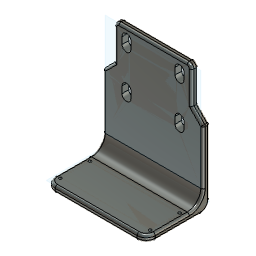
Polycase-Voltaic-Bracket v11 (Autodesk Fusion 360 design; units mm, degrees)
Autodesk Fusion 360 part; units mm, degrees
sketch "Sketch1" plane through (0, 0, 0) normal (0, 0, 1) x (1, 0, 0)
sketch "Sketch2" plane through (0, 0, 0) normal (0, 0, 1) x (1, 0, 0)
  line L0 (-101.7193, 55.502) -> (37.9807, 55.502)
  line L1 (37.9807, 55.502) -> (37.9807, -33.398)
  line L2 (37.9807, -33.398) -> (-101.7193, -33.398)
  line L3 (-101.7193, -33.398) -> (-101.7193, 55.502)
  dimension "d1" = 139.7
  dimension "d2" = 88.9
  constraint horizontal L0
  constraint vertical L1
  constraint horizontal L2
  constraint vertical L3
  measures "d1" distance of L0.start L0.end
  measures "d2" distance of L0.end L1.end
extrude "Extrude1" add sketch "Sketch2" along normal blind 9.525
sketch "Sketch3" plane through (0, 0, 9.525) normal (0, 0, 1) x (-1, 0, 0)
  line L0 (101.7193, 33.398) -> (-37.9807, 33.398)
  line L1 (-37.9807, 33.398) -> (-37.9807, -55.502)
  line L2 (-37.9807, -55.502) -> (101.7193, -55.502)
  line L3 (101.7193, -55.502) -> (101.7193, 33.398)
sketch "Sketch4" plane through (0, 0, 9.525) normal (0, 0, 1) x (-1, 0, 0)
  line L0 (-37.9807, -55.502) -> (101.7193, -55.502)
  line L1 (101.7193, -55.502) -> (101.7193, -45.977)
  line L2 (101.7193, -45.977) -> (-37.9807, -45.977)
  line L3 (-37.9807, -45.977) -> (-37.9807, -55.502)
  line L4 (101.7193, -55.502) -> (101.7193, 33.398)
  point P0 (-37.9807, -55.502)
  dimension "d5" = 9.525
  constraint horizontal L0
  constraint vertical L1
  constraint horizontal L2
  constraint vertical L3
  constraint coincident L1.end L4
  constraint coincident P0 L0.start
  measures "d5" distance of L0.end L1.end
extrude "Extrude2" add sketch "Sketch4" along normal blind 165.1
fillet "Fillet1" radius 19.05 1 edges at (-31.8693, 45.977, 9.525)
sketch "Sketch5" plane through (0, 0, 0) normal (0, 0, -1) x (1, 0, 0)
  line L0 (37.9807, 33.398) -> (-101.7193, 33.398)
  line L1 (-101.7193, 33.398) -> (-101.7193, -55.502)
  line L2 (-101.7193, -55.502) -> (37.9807, -55.502)
  line L3 (37.9807, -55.502) -> (37.9807, 33.398)
  line L4 (-94.5819, 33.398) -> (-94.5819, 20.698) construction
  line L5 (-94.5819, 20.698) -> (-101.7193, 20.698) construction
  line L6 (30.8433, 33.398) -> (30.8433, 20.698) construction
  line L7 (30.8433, 20.698) -> (37.9807, 20.698) construction
  line L8 (-94.5819, 20.698) -> (-94.5819, -20.577) construction
  line L9 (-94.5819, -20.577) -> (30.8433, -20.577) construction
  line L10 (30.8433, -20.577) -> (30.8433, 20.698) construction
  line L11 (-94.5819, 20.698) -> (30.8433, 20.698) construction
  circle A0 centre (-94.5819, 20.698) radius 1.905
  circle A1 centre (30.8433, 20.698) radius 1.905
  circle A2 centre (30.8433, -20.577) radius 1.905
  circle A3 centre (-94.5819, -20.577) radius 1.905
  dimension "d12" = 41.275
  dimension "d13" = 125.4252
  dimension "d14" = 3.81
  dimension "d15" = 12.7
  constraint coincident L0 L4.start
  constraint perpendicular L0 L4
  constraint coincident L1 L5.end
  constraint perpendicular L1 L5
  constraint coincident L0 L6.start
  constraint perpendicular L0 L6
  constraint coincident L3 L7.end
  constraint perpendicular L3 L7
  constraint collinear L5 L7
  constraint equal L5 L7
  constraint perpendicular L5 L8
  constraint perpendicular L6 L9
  constraint perpendicular L7 L10
  constraint coincident L4.end L5.start
  constraint coincident L6.end L7.start
  constraint coincident L9.end L10.start
  constraint coincident L8.end L9.start
  constraint equal A1 A2
  constraint equal A2 A3
  constraint equal A0 A3
  measures "d12" distance of L4.end L8.end
  measures "d13" distance of L4.end L6.end
  measures "d14" diameter of A0
  measures "d15" distance of L4.start L4.end
extrude "Extrude3" cut sketch "Sketch5" against normal through all contours A0 | A1 | A2 | A3
fillet "Fillet2" radius 12.7 2 edges at (37.9807, -33.398, 4.7625) (-101.7193, -33.398, 4.7625)
fillet "Fillet3" radius 3.175 18 edges at (37.9807, 17.402, 0) (34.2609, -29.6782, 0) (-31.8693, -33.398, 0) (-97.9996, -29.6782, 0) (-101.7193, 17.402, 0) (37.9807, 45.977, 101.6) (37.9807, 40.3974, 15.1046) (37.9807, 3.1145, 9.525) (34.2609, -29.6782, 9.525) (-31.8693, -33.398, 9.525) (-97.9996, -29.6782, 9.525) (-101.7193, 3.1145, 9.525) (-101.7193, 40.3974, 15.1046) (-101.7193, 45.977, 101.6) (-101.7193, 55.502, 87.3125) (-31.8693, 45.977, 174.625) (-31.8693, 55.502, 174.625) (37.9807, 55.502, 87.3125)
fillet "Fillet4" radius 12.7 3 edges at (-100.7894, 54.5721, 0.9299) (-31.8693, 55.502, 0) (37.0507, 54.5721, 0.9299)
sketch "Sketch6" plane through (0, 45.977, 0) normal (0, -1, 0) x (1, 0, 0)
  line L0 (34.8057, 28.575) -> (34.8057, 171.45)
  line L1 (34.8057, 171.45) -> (-98.5443, 171.45)
  line L2 (-98.5443, 171.45) -> (-98.5443, 28.575)
  line L3 (-98.5443, 28.575) -> (34.8057, 28.575)
fillet "Fillet5" radius 12.7 6 edges at (-100.7894, 54.5721, 173.6951) (-101.7193, 50.7395, 174.625) (-100.7894, 46.907, 173.6951) (37.0507, 46.907, 173.6951) (37.9807, 50.7395, 174.625) (37.0507, 54.5721, 173.6951)
sketch "Sketch7" plane through (0, 55.502, 0) normal (0, 1, 0) x (-1, 0, 0)
  arc A0 (-25.2807, 171.45) -> (-34.8057, 161.925) centre (-25.2807, 161.925) ccw
  line L0 (-34.8057, 161.925) -> (-34.8057, 12.7)
  line L1 (-34.8057, 12.7) -> (98.5443, 12.7)
  line L2 (98.5443, 12.7) -> (98.5443, 161.925)
  arc A1 (98.5443, 161.925) -> (89.0193, 171.45) centre (89.0193, 161.925) ccw
  line L3 (89.0193, 171.45) -> (-25.2807, 171.45)
  line L4 (-34.8057, 157.2) -> (-5.1407, 157.2) construction
  line L5 (-5.1407, 157.2) -> (-5.1407, 171.45) construction
  line L6 (68.8793, 171.45) -> (68.8793, 157.2) construction
  line L7 (68.8793, 157.2) -> (98.5443, 157.2) construction
  line L8 (1.1093, 157.2) -> (68.8793, 157.2) construction
  line L9 (-5.1407, 157.2) -> (-5.1407, 147.7) construction
  line L10 (68.8793, 157.2) -> (68.8793, 147.7) construction
  line L11 (-5.1407, 147.7) -> (1.1093, 147.7) construction
  line L12 (1.1093, 157.2) -> (-11.3907, 157.2) construction
  line L13 (-11.3907, 147.7001) -> (-11.3907, 157.2)
  line L14 (1.1093, 157.2) -> (1.1093, 147.7)
  arc A2 (1.1093, 157.2) -> (-11.3907, 157.2) centre (-5.1407, 157.2) ccw
  arc A3 (-11.3907, 147.7001) -> (1.1093, 147.7) centre (-5.1407, 147.7) ccw
  line L15 (62.6293, 157.2) -> (62.6293, 147.7)
  line L16 (75.1288, 147.62) -> (75.0405, 157.2)
  arc A4 (62.6293, 147.7) -> (75.1288, 147.62) centre (68.8793, 147.7) ccw
  arc A5 (75.0405, 157.2) -> (62.6293, 157.2) centre (68.8349, 157.9439) ccw
  line L17 (-5.1407, 147.7) -> (-5.1407, 97.7) construction
  line L18 (68.8793, 147.7) -> (68.8793, 97.7)
  line L19 (-5.1407, 97.7) -> (-5.1407, 88.2) construction
  line L20 (68.8793, 97.7) -> (68.8793, 88.2) construction
  line L21 (-5.1407, 88.2) -> (1.1093, 88.2) construction
  line L22 (1.1093, 97.7033) -> (1.1093, 88.2)
  line L23 (-11.3907, 88.1982) -> (-11.3907, 97.7)
  arc A6 (1.1093, 97.7033) -> (-11.3907, 97.7) centre (-5.1407, 97.7) ccw
  arc A7 (-11.3907, 88.1982) -> (1.1093, 88.2) centre (-5.1407, 88.2) ccw
  line L24 (68.8793, 97.7) -> (62.6293, 97.7) construction
  line L25 (62.6293, 97.7) -> (62.6293, 88.2)
  line L26 (68.8793, 97.7) -> (75.1293, 97.7) construction
  line L27 (75.1293, 97.7) -> (75.1293, 88.2)
  arc A8 (75.1293, 97.7) -> (62.6293, 97.7) centre (68.8793, 97.7) ccw
  arc A9 (62.6293, 88.2) -> (75.1293, 88.2) centre (68.8793, 88.2) ccw
  dimension "d25" = 74.02
  dimension "d26" = 14.25
  dimension "d27" = 12.5
  dimension "d28" = 23.75
  dimension "d29" = 9.5
  dimension "d30" = 12.5
  dimension "d33" = 6.25
  dimension "d34" = 50
  constraint coincident L0 L4.start
  constraint perpendicular L0 L4
  constraint coincident L3 L5.end
  constraint perpendicular L3 L5
  constraint coincident L3 L6.start
  constraint perpendicular L3 L6
  constraint coincident L2 L7.end
  constraint perpendicular L2 L7
  constraint equal L4 L7
  constraint equal L5 L6
  constraint coincident L4.end L5.start
  constraint perpendicular L4 L9
  constraint perpendicular L7 L10
  constraint equal L9 L10
  constraint coincident L9.end L11.start
  constraint coincident L10.end A4.centre
  constraint equal A3 A4
  constraint equal A2 A3
  constraint perpendicular L9 L11
  constraint coincident L4 L12.end
  constraint tangent L13 A2
  constraint coincident L8 L15.start
  constraint tangent L15 A4
  constraint perpendicular L8 L15
  constraint coincident L7 L16.end
  constraint perpendicular L11 L17
  constraint perpendicular L8 L18
  constraint equal L17 L18
  constraint coincident L17.end L19.start
  constraint coincident L18.end L20.start
  constraint parallel L17 L19
  constraint parallel L18 L20
  constraint equal L19 L20
  constraint coincident L19.end L21.start
  constraint coincident L20.end A9.centre
  constraint equal A6 A7
  constraint equal A6 A8
  constraint equal A8 A9
  constraint perpendicular L19 L21
  constraint tangent L22 A7
  constraint tangent L23 A6
  constraint perpendicular L21 L23
  constraint perpendicular L18 L24
  constraint tangent L25 A9
  constraint perpendicular L18 L26
  constraint tangent L27 A9
  constraint horizontal L8
  measures "d25" distance of L4.end L6.end
  measures "d26" distance of L4.end L5.end
  measures "d27" diameter of A2
  measures "d28" distance of L3 L9.end
  measures "d29" distance of L17.end L19.end
  measures "d30" diameter of A6
  measures "d33" radius of A5
  measures "d34" distance of L9.end L17.end
extrude "Extrude4" cut sketch "Sketch7" against normal through all contours L13 L14 A2 A3 | L15 L16 A4 A5 | L22 L23 A6 A7 | L25 L27 A8 A9
sketch "Sketch8" plane through (0, 45.977, 0) normal (0, -1, 0) x (1, 0, 0)
  line L0 (34.8057, 171.45) -> (-98.5443, 171.45)
  line L1 (-85.8443, 171.45) -> (-85.8443, 120.65)
  line L2 (-85.8443, 120.65) -> (-109.5291, 96.9652)
  line L3 (-109.5291, 96.9652) -> (-109.5291, 201.1527)
  line L4 (-109.5291, 201.1527) -> (45.7904, 201.1527)
  line L5 (45.7904, 201.1527) -> (45.7904, 96.9652)
  line L6 (45.7904, 96.9652) -> (22.1057, 120.65)
  line L7 (22.1057, 120.65) -> (22.1057, 171.45)
  line L8 (-98.5443, 171.45) -> (-98.5443, 28.575) construction
  line L9 (-98.5443, 145.4242) -> (-109.5291, 145.4242) construction
  line L10 (34.8057, 28.575) -> (34.8057, 171.45) construction
  line L11 (34.8057, 145.4242) -> (45.7904, 145.4242) construction
  line L12 (-98.5443, 145.4242) -> (-85.8443, 145.4242) construction
  line L13 (34.8057, 145.4242) -> (22.1057, 145.4242) construction
  dimension "d35" = 135
  dimension "d36" = 50.8
  dimension "d37" = 12.7
  constraint coincident L0 L1.start
  constraint perpendicular L0 L1
  constraint perpendicular L0 L3
  constraint perpendicular L3 L4
  constraint perpendicular L4 L5
  constraint coincident L0 L7.end
  constraint perpendicular L0 L7
  constraint equal L1 L7
  constraint equal L2 L6
  constraint equal L3 L5
  constraint coincident L8 L9.start
  constraint coincident L3 L9.end
  constraint perpendicular L3 L9
  constraint coincident L10 L11.start
  constraint coincident L5 L11.end
  constraint perpendicular L5 L11
  constraint collinear L9 L11
  constraint coincident L1 L12.end
  constraint perpendicular L1 L12
  constraint coincident L7 L13.end
  constraint perpendicular L7 L13
  constraint equal L12 L13
  measures "d35" angle of L1 L2
  measures "d36" distance of L1.start L1.end
  measures "d37" distance of L9.start L12.end
extrude "Extrude5" cut sketch "Sketch8" against normal through all
fillet "Fillet6" radius 3.175 16 edges at (22.1057, 45.977, 146.05) (28.4557, 55.502, 114.3) (37.0507, 54.5721, 105.7049) (37.9807, 50.7395, 104.775) (37.0507, 46.907, 105.7049) (28.4557, 45.977, 114.3) (-85.8443, 45.977, 146.05) (-92.1943, 45.977, 114.3) (-100.7894, 46.907, 105.7049) (-101.7193, 50.7395, 104.775) (-100.7894, 54.5721, 105.7049) (-92.1943, 55.502, 114.3) (22.1057, 55.502, 146.05) (-85.8443, 55.502, 146.05) (-31.8693, 55.502, 171.45) (-31.8693, 45.977, 171.45)
fillet "Fillet7" radius 6.35 6 edges at (-84.9144, 46.907, 170.5201) (-85.8443, 50.7395, 171.45) (-84.9144, 54.5721, 170.5201) (21.1757, 46.907, 170.5201) (22.1057, 50.7395, 171.45) (21.1757, 54.5721, 170.5201)
